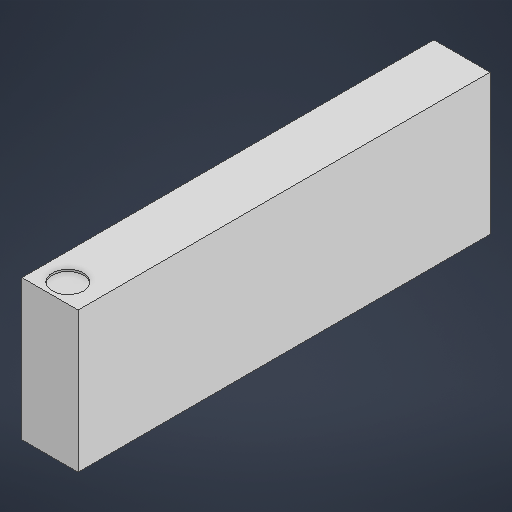
# Autodesk Inventor part: backbackmotorwall
Saved by Autodesk Inventor 2026.2 (Build 302298010, 298A)
## iProperties
Created: 2026-03-30
Part Number: backbackmotorwall
Material: Generic
Document SubType Name: Modeling
Designer: karol
Density: 1 g/cm^3
Appearance: Default
Author: karol
Autodesk Inventor part; units mm, degrees
ref_plane "YZ Plane" through (0, 0, 0) normal (1, 0, 0) x (0, 1, 0)
ref_plane "XZ Plane" through (0, 0, 0) normal (0, 1, 0) x (-1, 0, 0)
ref_plane "XY Plane" through (0, 0, 0) normal (0, 0, 1) x (1, 0, 0)
sketch "Sketch1" plane through (0, 0, 0) normal (0, 1, 0) x (-1, 0, 0)
  line L0 (0, 0) -> (3, 0)
  line L1 (3, 0) -> (3, -22)
  line L2 (3, -22) -> (0, -22)
  line L3 (0, -22) -> (0, 0)
  dimension "d0" = 3
  dimension "d1" = 22
  constraints: 8 end point, 2 parallel, 1 horizontal, 1 perpendicular
  measures "d0" distance of L1.end L2.end
  measures "d1" distance of L0.end L1.end
extrude "Extrusion1" add sketch "Sketch1" along normal blind 7.5
sketch "Sketch2" plane through (0, 7.5, 0) normal (0, 1, 0) x (1, 0, 0)
  circle A0 centre (-1.5727, 1.0248) radius 0.8357
  point P0 (0, 0)
  constraints: 1 centre point
extrude "Extrusion2" cut sketch "Sketch2" against normal blind 0.1
body "Solid1"
